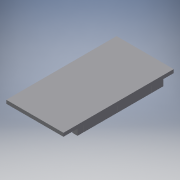
# Autodesk Inventor part: NodeMcu
Saved by Autodesk Inventor 2017 (Build 210142000, 142)
## iProperties
Created: 2020-04-05
Part Number: NodeMcu
Material: Generic
Document SubType Name: Modeling
Designer: LaNave
Density: 1 g/cm^3
Appearance: Default
Mass: 18.1298 g
Surface Area: 136.167 cm^2
Volume: 18.1298 cm^3
Author: LaNave
Autodesk Inventor part; units mm, degrees
ref_plane "YZ Plane" through (0, 0, 0) normal (1, 0, 0) x (0, 1, 0)
ref_plane "XZ Plane" through (0, 0, 0) normal (0, 1, 0) x (-1, 0, 0)
ref_plane "XY Plane" through (0, 0, 0) normal (0, 0, 1) x (1, 0, 0)
sketch "Sketch1" plane through (0, 0, 0) normal (0, 1, 0) x (-1, 0, 0)
  line L0 (0, 0) -> (50, 0)
  line L1 (50, 0) -> (50, 96.4)
  line L2 (50, 96.4) -> (0, 96.4)
  line L3 (0, 96.4) -> (0, 0)
  dimension "d0" = 96.4
  dimension "d1" = 50
  constraints: 8 end point, 2 parallel, 1 horizontal, 1 perpendicular
  measures "d0" distance of L1.end L0.end
  measures "d1" distance of L1.end L2.end
extrude "Extrusion1" add sketch "Sketch1" along normal blind 3
sketch "Sketch2" plane through (0, 0, 0) normal (0, -1, 0) x (1, 0, 0)
  line L0 (0, 0) -> (-50, 0) projected
  line L1 (-50, 96.4) -> (0, 96.4) projected
  line L2 (0, 0) -> (-4.6, 0)
  line L3 (-4.6, 0) -> (-4.6, 96.4)
  line L4 (-4.6, 96.4) -> (0, 96.4)
  line L5 (0, 96.4) -> (0, 0)
  line L6 (-45.3856, 0) -> (-49.9856, 0)
  line L7 (-49.9856, 0) -> (-49.9856, 96.2996)
  line L8 (-49.9856, 96.2996) -> (-45.3856, 96.2996)
  line L9 (-45.3856, 96.2996) -> (-45.3856, 0)
  dimension "d4" = 4.6
  dimension "d5" = 4.6
  constraints: 16 end point, 4 parallel, 2 horizontal, 2 perpendicular, 1 point on line
  measures "d4" distance of L3.end L4.end
  measures "d5" distance of L7.end L8.end
extrude "Extrusion2" add sketch "Sketch2" along normal blind 0.001
sketch "Sketch3" plane through (0, -0.001, 0) normal (0, -1, 0) x (1, 0, 0)
  line L0 (-4.6, 0) -> (0, 0) projected
  line L1 (-4.6, 96.4) -> (-4.6, 0) projected
  line L2 (-45.3048, 9.2015) -> (-49.9081, 9.2015)
  line L3 (-49.9081, 9.2015) -> (-49.9081, 14.1215)
  line L4 (-49.9081, 14.1215) -> (-45.3048, 14.1215)
  line L5 (-45.3048, 14.1215) -> (-45.3048, 9.2015)
  line L6 (0, 96.4) -> (0, 0) projected
  line L7 (-45.3048, 14.2015) -> (-49.9081, 14.2015)
  line L8 (-49.9081, 14.2015) -> (-49.9081, 19.1215)
  line L9 (-49.9081, 19.1215) -> (-45.3048, 19.1215)
  line L10 (-45.3048, 19.1215) -> (-45.3048, 14.2015)
  line L11 (-45.3048, 19.2015) -> (-49.9081, 19.2015)
  line L12 (-49.9081, 19.2015) -> (-49.9081, 24.1215)
  line L13 (-49.9081, 24.1215) -> (-45.3048, 24.1215)
  line L14 (-45.3048, 24.1215) -> (-45.3048, 19.2015)
  line L15 (-45.3048, 24.2015) -> (-49.9081, 24.2015)
  line L16 (-49.9081, 24.2015) -> (-49.9081, 29.1215)
  line L17 (-49.9081, 29.1215) -> (-45.3048, 29.1215)
  line L18 (-45.3048, 29.1215) -> (-45.3048, 24.2015)
  line L19 (-45.3048, 29.2015) -> (-49.9081, 29.2015)
  line L20 (-49.9081, 29.2015) -> (-49.9081, 34.1215)
  line L21 (-49.9081, 34.1215) -> (-45.3048, 34.1215)
  line L22 (-45.3048, 34.1215) -> (-45.3048, 29.2015)
  line L23 (-45.3048, 34.2015) -> (-49.9081, 34.2015)
  line L24 (-49.9081, 34.2015) -> (-49.9081, 39.1215)
  line L25 (-49.9081, 39.1215) -> (-45.3048, 39.1215)
  line L26 (-45.3048, 39.1215) -> (-45.3048, 34.2015)
  line L27 (-45.3048, 39.2015) -> (-49.9081, 39.2015)
  line L28 (-49.9081, 39.2015) -> (-49.9081, 44.1215)
  line L29 (-49.9081, 44.1215) -> (-45.3048, 44.1215)
  line L30 (-45.3048, 44.1215) -> (-45.3048, 39.2015)
  line L31 (-45.3048, 44.2015) -> (-49.9081, 44.2015)
  line L32 (-49.9081, 44.2015) -> (-49.9081, 49.1215)
  line L33 (-49.9081, 49.1215) -> (-45.3048, 49.1215)
  line L34 (-45.3048, 49.1215) -> (-45.3048, 44.2015)
  line L35 (-45.3048, 49.2015) -> (-49.9081, 49.2015)
  line L36 (-49.9081, 49.2015) -> (-49.9081, 54.1215)
  line L37 (-49.9081, 54.1215) -> (-45.3048, 54.1215)
  line L38 (-45.3048, 54.1215) -> (-45.3048, 49.2015)
  line L39 (-45.3048, 54.2015) -> (-49.9081, 54.2015)
  line L40 (-49.9081, 54.2015) -> (-49.9081, 59.1215)
  line L41 (-49.9081, 59.1215) -> (-45.3048, 59.1215)
  line L42 (-45.3048, 59.1215) -> (-45.3048, 54.2015)
  line L43 (-45.3048, 59.2015) -> (-49.9081, 59.2015)
  line L44 (-49.9081, 59.2015) -> (-49.9081, 64.1215)
  line L45 (-49.9081, 64.1215) -> (-45.3048, 64.1215)
  line L46 (-45.3048, 64.1215) -> (-45.3048, 59.2015)
  line L47 (-45.3048, 64.2015) -> (-49.9081, 64.2015)
  line L48 (-49.9081, 64.2015) -> (-49.9081, 69.1215)
  line L49 (-49.9081, 69.1215) -> (-45.3048, 69.1215)
  line L50 (-45.3048, 69.1215) -> (-45.3048, 64.2015)
  line L51 (-45.3048, 69.2015) -> (-49.9081, 69.2015)
  line L52 (-49.9081, 69.2015) -> (-49.9081, 74.1215)
  line L53 (-49.9081, 74.1215) -> (-45.3048, 74.1215)
  line L54 (-45.3048, 74.1215) -> (-45.3048, 69.2015)
  line L55 (-45.3048, 74.2015) -> (-49.9081, 74.2015)
  line L56 (-49.9081, 74.2015) -> (-49.9081, 79.1215)
  line L57 (-49.9081, 79.1215) -> (-45.3048, 79.1215)
  line L58 (-45.3048, 79.1215) -> (-45.3048, 74.2015)
  line L59 (-45.3048, 79.2015) -> (-49.9081, 79.2015)
  line L60 (-49.9081, 79.2015) -> (-49.9081, 84.1215)
  line L61 (-49.9081, 84.1215) -> (-45.3048, 84.1215)
  line L62 (-45.3048, 84.1215) -> (-45.3048, 79.2015)
  line L63 (-50, 0) -> (-50, 96.4) projected
  line L64 (-50, 9.2015) -> (-50, 96.4)
  line L65 (0, 9.2015) -> (-4.6032, 9.2015)
  line L66 (-4.6032, 9.2015) -> (-4.6032, 14.1215)
  line L67 (-4.6032, 14.1215) -> (0, 14.1215)
  line L68 (0, 14.1215) -> (0, 9.2015)
  line L69 (0, 14.2015) -> (-4.6032, 14.2015)
  line L70 (-4.6032, 14.2015) -> (-4.6032, 19.1215)
  line L71 (-4.6032, 19.1215) -> (0, 19.1215)
  line L72 (0, 19.1215) -> (0, 14.2015)
  line L73 (0, 19.2015) -> (-4.6032, 19.2015)
  line L74 (-4.6032, 19.2015) -> (-4.6032, 24.1215)
  line L75 (-4.6032, 24.1215) -> (0, 24.1215)
  line L76 (0, 24.1215) -> (0, 19.2015)
  line L77 (0, 24.2015) -> (-4.6032, 24.2015)
  line L78 (-4.6032, 24.2015) -> (-4.6032, 29.1215)
  line L79 (-4.6032, 29.1215) -> (0, 29.1215)
  line L80 (0, 29.1215) -> (0, 24.2015)
  line L81 (0, 29.2015) -> (-4.6032, 29.2015)
  line L82 (-4.6032, 29.2015) -> (-4.6032, 34.1215)
  line L83 (-4.6032, 34.1215) -> (0, 34.1215)
  line L84 (0, 34.1215) -> (0, 29.2015)
  line L85 (0, 34.2015) -> (-4.6032, 34.2015)
  line L86 (-4.6032, 34.2015) -> (-4.6032, 39.1215)
  line L87 (-4.6032, 39.1215) -> (0, 39.1215)
  line L88 (0, 39.1215) -> (0, 34.2015)
  line L89 (0, 39.2015) -> (-4.6032, 39.2015)
  line L90 (-4.6032, 39.2015) -> (-4.6032, 44.1215)
  line L91 (-4.6032, 44.1215) -> (0, 44.1215)
  line L92 (0, 44.1215) -> (0, 39.2015)
  line L93 (0, 44.2015) -> (-4.6032, 44.2015)
  line L94 (-4.6032, 44.2015) -> (-4.6032, 49.1215)
  line L95 (-4.6032, 49.1215) -> (0, 49.1215)
  line L96 (0, 49.1215) -> (0, 44.2015)
  line L97 (0, 49.2015) -> (-4.6032, 49.2015)
  line L98 (-4.6032, 49.2015) -> (-4.6032, 54.1215)
  line L99 (-4.6032, 54.1215) -> (0, 54.1215)
  line L100 (0, 54.1215) -> (0, 49.2015)
  line L101 (0, 54.2015) -> (-4.6032, 54.2015)
  line L102 (-4.6032, 54.2015) -> (-4.6032, 59.1215)
  line L103 (-4.6032, 59.1215) -> (0, 59.1215)
  line L104 (0, 59.1215) -> (0, 54.2015)
  line L105 (0, 59.2015) -> (-4.6032, 59.2015)
  line L106 (-4.6032, 59.2015) -> (-4.6032, 64.1215)
  line L107 (-4.6032, 64.1215) -> (0, 64.1215)
  line L108 (0, 64.1215) -> (0, 59.2015)
  line L109 (0, 64.2015) -> (-4.6032, 64.2015)
  line L110 (-4.6032, 64.2015) -> (-4.6032, 69.1215)
  line L111 (-4.6032, 69.1215) -> (0, 69.1215)
  line L112 (0, 69.1215) -> (0, 64.2015)
  line L113 (0, 69.2015) -> (-4.6032, 69.2015)
  line L114 (-4.6032, 69.2015) -> (-4.6032, 74.1215)
  line L115 (-4.6032, 74.1215) -> (0, 74.1215)
  line L116 (0, 74.1215) -> (0, 69.2015)
  line L117 (0, 74.2015) -> (-4.6032, 74.2015)
  line L118 (-4.6032, 74.2015) -> (-4.6032, 79.1215)
  line L119 (-4.6032, 79.1215) -> (0, 79.1215)
  line L120 (0, 79.1215) -> (0, 74.2015)
  line L121 (0, 79.2015) -> (-4.6032, 79.2015)
  line L122 (-4.6032, 79.2015) -> (-4.6032, 84.1215)
  line L123 (-4.6032, 84.1215) -> (0, 84.1215)
  line L124 (0, 84.1215) -> (0, 79.2015)
  point P0 (0, 9.2)
  point P1 (0, 14.2)
  point P2 (0, 19.2)
  point P3 (0, 24.2)
  point P4 (0, 29.2)
  point P5 (0, 34.2)
  point P6 (0, 39.2)
  point P7 (0, 44.2)
  point P8 (0, 49.2)
  point P9 (0, 54.2)
  point P10 (0, 59.2)
  point P11 (0, 64.2)
  point P12 (0, 69.2)
  point P13 (0, 74.2)
  point P14 (0, 79.2)
  point P15 (-4.6952, 9.2015)
  dimension "d13" = 5
  dimension "d36" = 5
  constraints: 186 end point, 4 parallel, 2 horizontal, 2 perpendicular, 2 point on line, 1 collinear, 1 vertical, 14 other
  measures "d13" distance of L3.end L8.end
  measures "d36" distance of L66.end L71.start
extrude "Extrusion3" add sketch "Sketch3" along normal blind 5.4 contours L65 L66 L67 L1 | L1 L67 L6 L65 | L69 L70 L71 L1 | L1 L71 L6 L69 | L73 L74 L75 L1 | L1 L75 L6 L73 | L77 L78 L79 L1 | L1 L79 L6 L77 | L81 L82 L83 L1 | L1 L83 L6 L81 | L85 L86 L87 L1 | L1 L87 L6 L85 | L89 L90 L91 L1 | L1 L91 L6 L89 | L93 L94 L95 L1 | L1 L95 L6 L93 | L97 L98 L99 L1 | L1 L99 L6 L97 | L101 L102 L103 L1 | L1 L103 L6 L101 | L105 L106 L107 L1 | L1 L107 L6 L105 | L109 L110 L111 L1 | L1 L111 L6 L109 | L113 L114 L115 L1 | L1 L115 L6 L113 | L117 L118 L119 L1 | L1 L119 L6 L117 | L121 L122 L123 L1 | L1 L123 L6 L121 | L2 L3 L4 L5 | L7 L8 L9 L10 | L11 L12 L13 L14 | L15 L16 L17 L18 | L19 L20 L21 L22 | L23 L24 L25 L26 | L27 L28 L29 L30 | L31 L32 L33 L34 | L35 L36 L37 L38 | L39 L40 L41 L42 | L43 L44 L45 L46 | L47 L48 L49 L50 | L51 L52 L53 L54 | L55 L56 L57 L58 | L59 L60 L61 L62
scale "Scale1" factors (0.5, 0.5, 0.5) then translate (-1.1508, -1.3505, 37.0607) bodies 1
body "Solid1"
